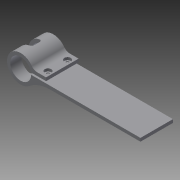
# Autodesk Inventor part: suporte-rodas
Saved by Autodesk Inventor 2015 (Build 190159000, 159)
## iProperties
Created: 2016-08-10
Part Number: suporte-rodas
Material: Ogólny
Document SubType Name: Modeling
Designer: EriveltonDell
Density: 1 g/cm^3
Appearance: Domyślna
Author: EriveltonDell
Autodesk Inventor part; units mm, degrees
ref_plane "YZ Plane" through (0, 0, 0) normal (1, 0, 0) x (0, 1, 0)
ref_plane "XZ Plane" through (0, 0, 0) normal (0, 1, 0) x (-1, 0, 0)
ref_plane "XY Plane" through (0, 0, 0) normal (0, 0, 1) x (1, 0, 0)
sketch "Sketch1" plane through (0, 0, 0) normal (0, 1, 0) x (-1, 0, 0)
  arc A0 (-16, 0) -> (-15.7162, 3) centre (0, 0) ccw
  arc A1 (-13.2802, -16.2676) -> (-17.0973, 12.1935) centre (0, 0) ccw
  line L0 (-16, 0) -> (-184, 0)
  line L1 (-184, 0) -> (-184, -5)
  line L2 (-184, -5) -> (-44.8999, -5)
  arc A2 (-13.2802, -16.2676) -> (-44.8999, -5) centre (-44.8999, -55) ccw
  line L3 (-39, 8) -> (-39, 3)
  line L4 (0, 0) -> (0, 3)
  line L5 (-15.7162, 3) -> (-39, 3)
  line L6 (-39, 3) -> (-39, 8)
  line L7 (-39, 8) -> (-25.2389, 8)
  arc A3 (-25.2389, 8) -> (-17.0973, 12.1935) centre (-25.2389, 18) ccw
  point P0 (-20.3961, -5)
  point P1 (-19.4165, 8)
  dimension "d0" = 32
  dimension "d1" = 42
  dimension "d2" = 168
  dimension "d3" = 5
  dimension "d4" = 50
  dimension "d7" = 3
  dimension "d8" = 39
  dimension "d9" = 5
  dimension "d10" = 3
  dimension "d11" = 39
  dimension "d12" = 10
  constraints: 16 end point, 10 point on circle, 4 centre point, 4 perpendicular, 4 tangent, 2 coincident, 2 point on line, 1 horizontal, 1 vertical
  measures "d0" diameter of A0
  measures "d1" diameter of A1
  measures "d2" distance of L0.start L0.end
  measures "d3" distance of L0.end L1.end
  measures "d4" radius of A2
  measures "d7" distance of L4.start L4.end
  measures "d8" distance of L3.end L4.end
  measures "d9" distance of L3.end L3.start
  measures "d10" distance from line of L0 L5.start
  measures "d11" distance from line of L4.start L3
  measures "d12" radius of A3
extrude "Extrusion1" add sketch "Sketch1" along normal blind 50
hole "Hole1" at (32, 10, 8) direction (0, 0, -1) diameter 5.5 end through all counterbore diameter 10 counterbore depth 4
hole "Hole2" at (32, 40, 8) direction (0, 0, -1) diameter 5.5 end through all counterbore diameter 10 counterbore depth 4
sketch "Sketch2" plane through (0, 0, 0) normal (0, 0, 1) x (1, 0, 0)
  line L0 (0, 0) -> (0, 17)
  line L1 (-4, 17) -> (-21, 17)
  line L2 (-21, 17) -> (-21, 33)
  line L3 (-21, 33) -> (-4, 33)
  line L4 (0, 29) -> (0, 21)
  arc A0 (-4, 17) -> (0, 21) centre (-4, 21) ccw
  arc A1 (0, 29) -> (-4, 33) centre (-4, 29) ccw
  point P0 (0, 33)
  dimension "d33" = 17
  dimension "d34" = 21
  dimension "d35" = 16
  dimension "d36" = 21
  dimension "d37" = 4
  constraints: 10 end point, 5 point on line, 4 point on circle, 4 tangent, 2 centre point, 2 perpendicular, 1 collinear, 1 equal radius, 1 vertical
  measures "d33" distance of L0.start L0.end
  measures "d34" distance of L0.end L1.end
  measures "d35" distance of L1.end L2.end
  measures "d36" distance of L2.end point (0, 33)
  measures "d37" radius of A0
extrude "Extrusion2" cut sketch "Sketch2" along normal mid plane 50
body "Solid1"
